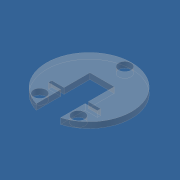
# Autodesk Inventor part: S1702_couverclerailressort
Saved by Autodesk Inventor 2015 SP2 (Build 190223200, 223)
## iProperties
Created: 2017-10-31
Part Number: S1702_couverclerailressort
Project: S1701_Circuit_Course_Manette
Material: Plastique PMMA
Description: Plaque Rail Ressort
Document SubType Name: Modeling
Designer: Benoit.CURCHOD2
Authority: Ø44x3
Density: 1.188 g/cm^3
Appearance: Transparent - Clair
Mass: 3.43675 g
Surface Area: 30.326 cm^2
Volume: 2.89288 cm^3
Material number: ---
Author: Benoit.CURCHOD2
Autodesk Inventor part; units mm, degrees
ref_plane "Plan YZ" through (0, 0, 0) normal (1, 0, 0) x (0, 1, 0)
ref_plane "Plan XZ" through (0, 0, 0) normal (0, 1, 0) x (-1, 0, 0)
ref_plane "Plan XY" through (0, 0, 0) normal (0, 0, 1) x (1, 0, 0)
sketch "Esquisse1" plane through (0, 0, 0) normal (0, 0, 1) x (1, 0, 0)
  arc A0 (6.3, -21.0787) -> (-6.3, -21.0787) centre (0, 0) ccw
  line L0 (-6.3, 6.7) -> (6.3, 6.7)
  line L1 (-6.3, -6.7) -> (-12.65, -6.7)
  line L2 (-12.65, -8.4) -> (-12.65, -6.7)
  line L3 (-6.3, -8.4) -> (-12.65, -8.4)
  line L4 (6.3, -6.7) -> (12.65, -6.7)
  line L5 (12.65, -6.7) -> (12.65, -8.4)
  line L6 (12.65, -8.4) -> (6.3, -8.4)
  line L7 (-30.8, 0) -> (30.8, 0) construction
  line L8 (0, -29.7044) -> (0, 30.6757) construction
  line L9 (-6.3, -21.0787) -> (-6.3, -8.4)
  line L10 (-6.3, -6.7) -> (-6.3, 6.7)
  line L11 (6.3, -8.4) -> (6.3, -21.0787)
  line L12 (6.3, -21.0787) -> (6.3, -8.4) construction
  line L13 (6.3, -21.0787) -> (6.3, -8.4)
  line L14 (6.3, -6.7) -> (6.3, 6.7)
  dimension "d0" = 44
  dimension "d47" = 1.7
  dimension "d49" = 6.35
  dimension "d52" = 12.6
  dimension "d55" = 13.4
  dimension "d56" = 6.7
  constraints: 26 end point, 3 horizontal, 3 vertical, 2 coincident, 2 parallel, 2 point on circle, 1 centre point, 1 collinear, 1 perpendicular, 5 other
  measures "d0" diameter of A0
  measures "d47" distance of L2.start L1.end
  measures "d49" distance of L3.start L2.start
  measures "d52" distance of L0.start L0.end
  measures "d55" distance of L4.start L0.end
  measures "d56" distance between parallel lines of L7 L1
extrude "Extrusion1" add sketch "Esquisse1" along normal blind 3
sketch "Esquisse7" plane through (0, 0, 3) normal (0, 0, 1) x (1, 0, 0)
  circle A0 centre (0, 18.5) radius 3.25
  circle A1 centre (10, -15.5644) radius 3.25
  circle A2 centre (-10, -15.5644) radius 3.25
  line L0 (0, -29.6944) -> (0, 30.6157) construction
  circle A3 centre (0, 0) radius 18.5 construction
  dimension "d23" = 6.5
  dimension "d34" = 20
  dimension "d51" = 37
  constraints: 4 centre point, 2 equal radius, 2 point on circle, 1 coincident, 1 point on line, 1 symmetric about line
  measures "d23" diameter of A0
  measures "d34" distance of A1.centre A2.centre
  measures "d51" diameter of A3
extrude "Extrusion5" cut sketch "Esquisse7" against normal through all
